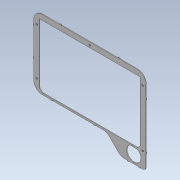
# Autodesk Inventor part: Лицевой лист
Saved by Autodesk Inventor 2021.2 (Build 252289000, 289)
## iProperties
Created: 2022-11-29
Part Number: Лицевой лист
Material: Типовые
Document SubType Name: ЛистМат
Designer: Voodoo
Density: 1 g/cm^3
Sheet Metal Rule: По умолчанию_мм
Appearance: По умолчанию
Mass: 42.3344 g
Surface Area: 479.036 cm^2
Volume: 42.3344 cm^3
Flat Pattern Width: 29.78 cm
Flat Pattern Length: 39.68 cm
Flat Pattern Area: 1181.67 cm^2
Sheet Metal Width: 297,800 мм
Sheet Metal Length: 396,800 мм
Sheet Metal Area: 118167,040 мм^2
Author: Voodoo
Autodesk Inventor part; units mm, degrees
ref_plane "YZ Plane" through (0, 0, 0) normal (1, 0, 0) x (0, 1, 0)
ref_plane "XZ Plane" through (0, 0, 0) normal (0, 1, 0) x (-1, 0, 0)
ref_plane "XY Plane" through (0, 0, 0) normal (0, 0, 1) x (1, 0, 0)
sketch "Эскиз6" plane through (0, 0, 2) normal (0, 0, 1) x (1, 0, 0)
  line L0 (-177, -106.1) -> (-177, 103.9)
  line L1 (-177, 103.9) -> (177, 103.9)
  line L2 (177, 103.9) -> (177, -106.1)
  line L3 (177, -106.1) -> (167, -116.1)
  line L4 (167, -116.1) -> (-167, -116.1)
  line L5 (-167, -116.1) -> (-177, -106.1)
  arc A0 (196.4, 92) -> (166.5, 121.9) centre (166.5, 92) ccw
  line L6 (-166.5, 121.9) -> (166.5, 121.9)
  arc A1 (-166.5, 121.9) -> (-196.4, 92) centre (-166.5, 92) ccw
  line L7 (-196.4, -92) -> (-196.4, 92)
  arc A2 (-196.4, -92) -> (-166.5, -121.9) centre (-166.5, -92) ccw
  line L8 (46.0736, -121.9) -> (-166.5, -121.9)
  arc A3 (68.7717, -131.3019) -> (46.0736, -121.9) centre (46.0736, -154) ccw
  line L9 (101.1981, -163.7283) -> (68.7717, -131.3019)
  arc A4 (101.1981, -163.7283) -> (120.9264, -171.9) centre (120.9264, -144) ccw
  line L10 (186.5, -171.9) -> (120.9264, -171.9)
  arc A5 (186.5, -171.9) -> (196.4, -162) centre (186.5, -162) ccw
  line L11 (196.4, 92) -> (196.4, -162)
  circle A6 centre (154.4, -141.9) radius 25
  line L12 (188.45, -115.4278) -> (188.45, -118.3722)
  line L13 (188.45, -118.3722) -> (185.9, -119.8445)
  line L14 (185.9, -119.8445) -> (183.35, -118.3722)
  line L15 (183.35, -118.3722) -> (183.35, -115.4278)
  line L16 (183.35, -115.4278) -> (185.9, -113.9555)
  line L17 (185.9, -113.9555) -> (188.45, -115.4278)
  line L18 (2.55, 112.8722) -> (2.55, 109.9278)
  line L19 (2.55, 109.9278) -> (0, 108.4555)
  line L20 (0, 108.4555) -> (-2.55, 109.9278)
  line L21 (-2.55, 109.9278) -> (-2.55, 112.8722)
  line L22 (-2.55, 112.8722) -> (0, 114.3445)
  line L23 (0, 114.3445) -> (2.55, 112.8722)
  line L24 (-183.35, 83.3722) -> (-183.35, 80.4278)
  line L25 (-183.35, 80.4278) -> (-185.9, 78.9555)
  line L26 (-185.9, 78.9555) -> (-188.45, 80.4278)
  line L27 (-188.45, 80.4278) -> (-188.45, 83.3722)
  line L28 (-188.45, 83.3722) -> (-185.9, 84.8445)
  line L29 (-185.9, 84.8445) -> (-183.35, 83.3722)
  line L30 (188.45, 83.3722) -> (188.45, 80.4278)
  line L31 (188.45, 80.4278) -> (185.9, 78.9555)
  line L32 (185.9, 78.9555) -> (183.35, 80.4278)
  line L33 (183.35, 80.4278) -> (183.35, 83.3722)
  line L34 (183.35, 83.3722) -> (185.9, 84.8445)
  line L35 (185.9, 84.8445) -> (188.45, 83.3722)
  line L36 (-183.35, -80.4278) -> (-183.35, -83.3722)
  line L37 (-183.35, -83.3722) -> (-185.9, -84.8445)
  line L38 (-185.9, -84.8445) -> (-188.45, -83.3722)
  line L39 (-188.45, -83.3722) -> (-188.45, -80.4278)
  line L40 (-188.45, -80.4278) -> (-185.9, -78.9555)
  line L41 (-185.9, -78.9555) -> (-183.35, -80.4278)
  line L42 (140.5306, -121.1) -> (168.2694, -121.1)
  point P0 (0, 0)
  dimension "d75" = 5
  measures "d75" distance between parallel lines of L4 L42
sketch "Эскиз7" plane through (0, 0, 0) normal (0, 0, -1) x (-1, 0, 0)
  line L0 (177, 103.9) -> (177, -106.1)
  line L1 (177, -106.1) -> (167, -116.1)
  line L2 (167, -116.1) -> (-167, -116.1)
  line L3 (-167, -116.1) -> (-177, -106.1)
  line L4 (-177, -106.1) -> (-177, 103.9)
  line L5 (-177, 103.9) -> (177, 103.9)
  line L6 (166.5, 121.9) -> (-166.5, 121.9)
  arc A0 (-166.5, 121.9) -> (-196.4, 92) centre (-166.5, 92) ccw
  line L7 (-196.4, 92) -> (-196.4, -162)
  arc A1 (-196.4, -162) -> (-186.5, -171.9) centre (-186.5, -162) ccw
  line L8 (-186.5, -171.9) -> (-120.9264, -171.9)
  arc A2 (-120.9264, -171.9) -> (-101.1981, -163.7283) centre (-120.9264, -144) ccw
  line L9 (-101.1981, -163.7283) -> (-68.7717, -131.3019)
  arc A3 (-46.0736, -121.9) -> (-68.7717, -131.3019) centre (-46.0736, -154) ccw
  line L10 (-46.0736, -121.9) -> (166.5, -121.9)
  arc A4 (166.5, -121.9) -> (196.4, -92) centre (166.5, -92) ccw
  line L11 (196.4, -92) -> (196.4, 92)
  arc A5 (196.4, 92) -> (166.5, 121.9) centre (166.5, 92) ccw
  arc A6 (-168.2694, -121.1) -> (-140.5306, -121.1) centre (-154.4, -141.9) ccw
  line L12 (-140.5306, -121.1) -> (-168.2694, -121.1)
  line L13 (-188.45, -118.3722) -> (-188.45, -115.4278)
  line L14 (-188.45, -115.4278) -> (-185.9, -113.9555)
  line L15 (-185.9, -113.9555) -> (-183.35, -115.4278)
  line L16 (-183.35, -115.4278) -> (-183.35, -118.3722)
  line L17 (-183.35, -118.3722) -> (-185.9, -119.8445)
  line L18 (-185.9, -119.8445) -> (-188.45, -118.3722)
  line L19 (-2.55, 109.9278) -> (-2.55, 112.8722)
  line L20 (-2.55, 112.8722) -> (0, 114.3445)
  line L21 (0, 114.3445) -> (2.55, 112.8722)
  line L22 (2.55, 112.8722) -> (2.55, 109.9278)
  line L23 (2.55, 109.9278) -> (0, 108.4555)
  line L24 (0, 108.4555) -> (-2.55, 109.9278)
  line L25 (183.35, 80.4278) -> (183.35, 83.3722)
  line L26 (183.35, 83.3722) -> (185.9, 84.8445)
  line L27 (185.9, 84.8445) -> (188.45, 83.3722)
  line L28 (188.45, 83.3722) -> (188.45, 80.4278)
  line L29 (188.45, 80.4278) -> (185.9, 78.9555)
  line L30 (185.9, 78.9555) -> (183.35, 80.4278)
  line L31 (-188.45, 80.4278) -> (-188.45, 83.3722)
  line L32 (-188.45, 83.3722) -> (-185.9, 84.8445)
  line L33 (-185.9, 84.8445) -> (-183.35, 83.3722)
  line L34 (-183.35, 83.3722) -> (-183.35, 80.4278)
  line L35 (-183.35, 80.4278) -> (-185.9, 78.9555)
  line L36 (-185.9, 78.9555) -> (-188.45, 80.4278)
  line L37 (183.35, -83.3722) -> (183.35, -80.4278)
  line L38 (183.35, -80.4278) -> (185.9, -78.9555)
  line L39 (185.9, -78.9555) -> (188.45, -80.4278)
  line L40 (188.45, -80.4278) -> (188.45, -83.3722)
  line L41 (188.45, -83.3722) -> (185.9, -84.8445)
  line L42 (185.9, -84.8445) -> (183.35, -83.3722)
  line L43 (-105, 121.9) -> (-100, 121.9)
  line L44 (-100, 121.9) -> (-100, 123.9)
  line L45 (-100, 123.9) -> (-105, 123.9)
  line L46 (-105, 123.9) -> (-105, 121.9)
  line L47 (100, 121.9) -> (105, 121.9)
  line L48 (105, 121.9) -> (105, 123.9)
  line L49 (105, 123.9) -> (100, 123.9)
  line L50 (100, 123.9) -> (100, 121.9)
  line L51 (0, 103.9) -> (0, 81.7755) construction
  line L52 (-196.4, 50) -> (-198.4, 50)
  line L53 (-198.4, 50) -> (-198.4, 45)
  line L54 (-198.4, 45) -> (-196.4, 45)
  line L55 (-196.4, 45) -> (-196.4, 50)
  line L56 (-196.4, -115) -> (-198.4, -115)
  line L57 (-198.4, -115) -> (-198.4, -120)
  line L58 (-198.4, -120) -> (-196.4, -120)
  line L59 (-196.4, -120) -> (-196.4, -115)
  line L60 (-176.4, -171.9) -> (-171.4, -171.9)
  line L61 (-171.4, -171.9) -> (-171.4, -173.9)
  line L62 (-171.4, -173.9) -> (-176.4, -173.9)
  line L63 (-176.4, -173.9) -> (-176.4, -171.9)
  line L64 (-18.6, -121.9) -> (-13.6, -121.9)
  line L65 (-13.6, -121.9) -> (-13.6, -123.9)
  line L66 (-13.6, -123.9) -> (-18.6, -123.9)
  line L67 (-18.6, -123.9) -> (-18.6, -121.9)
  line L68 (131.4, -121.9) -> (136.4, -121.9)
  line L69 (136.4, -121.9) -> (136.4, -123.9)
  line L70 (136.4, -123.9) -> (131.4, -123.9)
  line L71 (131.4, -123.9) -> (131.4, -121.9)
  line L72 (196.4, -28.1) -> (198.4, -28.1)
  line L73 (198.4, -28.1) -> (198.4, -23.1)
  line L74 (198.4, -23.1) -> (196.4, -23.1)
  line L75 (196.4, -23.1) -> (196.4, -28.1)
  line L76 (196.4, 76.9) -> (198.4, 76.9)
  line L77 (198.4, 76.9) -> (198.4, 71.9)
  line L78 (198.4, 71.9) -> (196.4, 71.9)
  line L79 (196.4, 71.9) -> (196.4, 76.9)
  line L80 (-196.4, -35) -> (-297.2205, -35)
  line L81 (-131.4, -171.9) -> (-136.4, -171.9)
  line L82 (-136.4, -171.9) -> (-136.4, -173.9)
  line L83 (-136.4, -173.9) -> (-131.4, -173.9)
  line L84 (-131.4, -173.9) -> (-131.4, -171.9)
  point P0 (0, 0)
  dimension "d81" = 5
  dimension "d82" = 2
  dimension "d83" = 5
  dimension "d84" = 2
  dimension "d85" = 100
  dimension "d86" = 100
  dimension "d87" = 2
  dimension "d88" = 5
  dimension "d89" = 2
  dimension "d90" = 5
  dimension "d91" = 5
  dimension "d92" = 2
  dimension "d93" = 5
  dimension "d94" = 2
  dimension "d95" = 5
  dimension "d96" = 2
  dimension "d97" = 2
  dimension "d98" = 5
  dimension "d99" = 2
  dimension "d100" = 5
  dimension "d101" = 80
  dimension "d102" = 80
  dimension "d103" = 20
  dimension "d104" = 60
  dimension "d105" = 150
  dimension "d106" = 45
  dimension "d107" = 100
  dimension "d113" = 5
  dimension "d114" = 2
  dimension "d115" = 40
  measures "d81" distance of L44.end L45.end
  measures "d82" distance of L45.end L43.start
  measures "d83" distance of L48.end L49.end
  measures "d84" distance of L49.end L47.start
  measures "d85" distance between parallel lines of L50 L51
  measures "d86" horizontal distance of L51.start L44.end
  measures "d87" distance of L54.end L53.end
  measures "d88" distance of L53.end L52.end
  measures "d89" distance of L58.end L57.end
  measures "d90" distance of L57.end L56.end
  measures "d91" distance of L61.end L62.end
  measures "d92" distance of L60.end L61.end
  measures "d93" distance of L65.end L66.end
  measures "d94" distance of L64.end L65.end
  measures "d95" distance of L69.end L70.end
  measures "d96" distance of L68.end L69.end
  measures "d97" distance of L74.end L73.end
  measures "d98" distance of L73.end L72.end
  measures "d99" distance of L77.end L78.end
  measures "d100" distance of L76.end L77.end
  measures "d101" distance between parallel lines of L56 L80
  measures "d102" distance from line of L54.end L80
  measures "d103" distance from line of L62.end L7
  measures "d104" distance from line of L69.end L11
  measures "d105" distance of L65.end L69.end
  measures "d106" distance from line of L76.end L6
  measures "d107" distance of L74.end L76.start
  measures "d113" distance of L83.end L82.end
  measures "d114" distance of L82.end L81.end
  measures "d115" distance from line of L63 L82.end
sketch "Эскиз1" plane through (0, 0, 0) normal (0, 0, 1) x (1, 0, 0)
  line L0 (-166.5, -124) -> (46.0736, -124)
  line L1 (198.5, -124) -> (198.5, 92)
  line L2 (166.5, 124) -> (-166.5, 124)
  line L3 (-198.5, 92) -> (-198.5, -92)
  line L4 (-198.5, -124) -> (198.5, 124) construction
  line L5 (198.5, -124) -> (-198.5, 124) construction
  arc A0 (-166.5, 124) -> (-198.5, 92) centre (-166.5, 92) ccw
  arc A1 (198.5, 92) -> (166.5, 124) centre (166.5, 92) ccw
  arc A2 (-198.5, -92) -> (-166.5, -124) centre (-166.5, -92) ccw
  line L6 (198.5, -124) -> (198.5, -162)
  line L7 (186.5, -174) -> (120.9264, -174)
  line L8 (99.7132, -165.2132) -> (67.2868, -132.7868)
  arc A3 (186.5, -174) -> (198.5, -162) centre (186.5, -162) ccw
  arc A4 (99.7132, -165.2132) -> (120.9264, -174) centre (120.9264, -144) ccw
  arc A5 (67.2868, -132.7868) -> (46.0736, -124) centre (46.0736, -154) ccw
  line L9 (-166.5, 121.9) -> (166.5, 121.9)
  arc A6 (196.4, 92) -> (166.5, 121.9) centre (166.5, 92) ccw
  line L10 (196.4, 92) -> (196.4, -145)
  line L11 (196.4, -145) -> (196.4, -162)
  arc A7 (186.5, -171.9) -> (196.4, -162) centre (186.5, -162) ccw
  line L12 (186.5, -171.9) -> (120.9264, -171.9)
  arc A8 (101.1981, -163.7283) -> (120.9264, -171.9) centre (120.9264, -144) ccw
  line L13 (101.1981, -163.7283) -> (68.7717, -131.3019)
  arc A9 (68.7717, -131.3019) -> (46.0736, -121.9) centre (46.0736, -154) ccw
  line L14 (46.0736, -121.9) -> (-166.5, -121.9)
  arc A10 (-196.4, -92) -> (-166.5, -121.9) centre (-166.5, -92) ccw
  line L15 (-196.4, -92) -> (-196.4, 92)
  arc A11 (-166.5, 121.9) -> (-196.4, 92) centre (-166.5, 92) ccw
  point P0 (0, 0)
  point P1 (198.5, -174)
  point P2 (108.5, -174)
  dimension "d2" = 397
  dimension "d3" = 248
  dimension "d4" = 32
  dimension "d5" = 298
  dimension "d6" = 12
  dimension "d7" = 50
  dimension "d8" = 90
  dimension "d9" = 135
  dimension "d10" = 30
  dimension "d11" = 2.1
  constraints: 32 end point, 24 point on circle, 12 centre point, 12 point on line, 12 tangent, 4 parallel, 4 perpendicular, 3 equal radius, 2 midpoint, 1 horizontal, 12 other
  measures "d2" distance of L5.end L4.end
  measures "d3" distance of L4.end L1.start
  measures "d4" radius of A0
  measures "d5" distance between parallel lines of L7 L2
  measures "d6" radius of A3
  measures "d7" distance between parallel lines of L0 L7
  measures "d8" distance from line of L6 point (108.5, -174)
  measures "d9" angle of L0 L8
  measures "d10" radius of A4
  measures "d11" distance between parallel lines of L2 L9
extrude "Пластина1" add sketch "Эскиз1" along normal blind 2 contours L9 A6 L10 L11 A7 L12 A8 L13 A9 L14 A10 L15 A11
sketch "Эскиз3" plane through (0, 0, 0) normal (0, 0, -1) x (-1, 0, 0)
  line L0 (166.5, 121.9) -> (-166.5, 121.9) projected
  arc A0 (-166.5, 121.9) -> (-196.4, 92) centre (-166.5, 92) ccw projected
  line L1 (-196.4, 92) -> (-196.4, -162) projected
  arc A1 (-196.4, -162) -> (-186.5, -171.9) centre (-186.5, -162) ccw projected
  line L2 (-186.5, -171.9) -> (-120.9264, -171.9) projected
  arc A2 (-120.9264, -171.9) -> (-101.1981, -163.7283) centre (-120.9264, -144) ccw projected
  line L3 (-101.1981, -163.7283) -> (-68.7717, -131.3019) projected
  arc A3 (-46.0736, -121.9) -> (-68.7717, -131.3019) centre (-46.0736, -154) ccw projected
  line L4 (-46.0736, -121.9) -> (166.5, -121.9) projected
  arc A4 (166.5, -121.9) -> (196.4, -92) centre (166.5, -92) ccw projected
  line L5 (196.4, -92) -> (196.4, 92) projected
  arc A5 (196.4, 92) -> (166.5, 121.9) centre (166.5, 92) ccw projected
  circle A6 centre (-154.4, -141.9) radius 25
  point P0 (0, 0)
  dimension "d19" = 50
  dimension "d20" = 30
  dimension "d21" = 42
  constraints: 1 centre point
  measures "d19" diameter of A6
  measures "d20" distance from line of A6.centre L2
  measures "d21" distance from line of A6.centre L1
extrude "Вырез2" cut sketch "Эскиз3" against normal blind 2 contours A6
sketch "Эскиз4" plane through (0, 0, 2) normal (0, 0, 1) x (1, 0, 0)
  circle A0 centre (154.4, -141.9) radius 25 projected
  arc A1 (196.4, 92) -> (166.5, 121.9) centre (166.5, 92) ccw projected
  line L0 (-166.5, 121.9) -> (166.5, 121.9) projected
  arc A2 (-166.5, 121.9) -> (-196.4, 92) centre (-166.5, 92) ccw projected
  line L1 (-196.4, -92) -> (-196.4, 92) projected
  arc A3 (-196.4, -92) -> (-166.5, -121.9) centre (-166.5, -92) ccw projected
  line L2 (46.0736, -121.9) -> (-166.5, -121.9) projected
  arc A4 (68.7717, -131.3019) -> (46.0736, -121.9) centre (46.0736, -154) ccw projected
  line L3 (101.1981, -163.7283) -> (68.7717, -131.3019) projected
  arc A5 (101.1981, -163.7283) -> (120.9264, -171.9) centre (120.9264, -144) ccw projected
  line L4 (186.5, -171.9) -> (120.9264, -171.9) projected
  arc A6 (186.5, -171.9) -> (196.4, -162) centre (186.5, -162) ccw projected
  line L5 (196.4, 92) -> (196.4, -162) projected
  circle A7 centre (-185.9, -81.9) radius 2.1
  circle A8 centre (-185.9, 81.9) radius 2.1
  circle A9 centre (0, 111.4) radius 2.1
  circle A10 centre (185.9, 81.9) radius 2.1
  circle A11 centre (185.9, -116.9) radius 2.1
  line L6 (-183.35, 80.4278) -> (-185.9, 78.9555)
  line L7 (-185.9, 78.9555) -> (-188.45, 80.4278)
  line L8 (-188.45, 80.4278) -> (-188.45, 83.3722)
  line L9 (-188.45, 83.3722) -> (-185.9, 84.8445)
  line L10 (-185.9, 84.8445) -> (-183.35, 83.3722)
  line L11 (-183.35, 83.3722) -> (-183.35, 80.4278)
  line L12 (2.55, 109.9278) -> (0, 108.4555)
  line L13 (0, 108.4555) -> (-2.55, 109.9278)
  line L14 (-2.55, 109.9278) -> (-2.55, 112.8722)
  line L15 (-2.55, 112.8722) -> (0, 114.3445)
  line L16 (0, 114.3445) -> (2.55, 112.8722)
  line L17 (2.55, 112.8722) -> (2.55, 109.9278)
  line L18 (188.45, 80.4278) -> (185.9, 78.9555)
  line L19 (185.9, 78.9555) -> (183.35, 80.4278)
  line L20 (183.35, 80.4278) -> (183.35, 83.3722)
  line L21 (183.35, 83.3722) -> (185.9, 84.8445)
  line L22 (185.9, 84.8445) -> (188.45, 83.3722)
  line L23 (188.45, 83.3722) -> (188.45, 80.4278)
  line L24 (188.45, -118.3722) -> (185.9, -119.8445)
  line L25 (185.9, -119.8445) -> (183.35, -118.3722)
  line L26 (183.35, -118.3722) -> (183.35, -115.4278)
  line L27 (183.35, -115.4278) -> (185.9, -113.9555)
  line L28 (185.9, -113.9555) -> (188.45, -115.4278)
  line L29 (188.45, -115.4278) -> (188.45, -118.3722)
  line L30 (-183.35, -83.3722) -> (-185.9, -84.8445)
  line L31 (-185.9, -84.8445) -> (-188.45, -83.3722)
  line L32 (-188.45, -83.3722) -> (-188.45, -80.4278)
  line L33 (-188.45, -80.4278) -> (-185.9, -78.9555)
  line L34 (-185.9, -78.9555) -> (-183.35, -80.4278)
  line L35 (-183.35, -80.4278) -> (-183.35, -83.3722)
  point P0 (0, 0)
  point P1 (0, 121.9)
  dimension "d34" = 4.2
  dimension "d36" = 4.2
  dimension "d37" = 4.2
  dimension "d38" = 4.2
  dimension "d52" = 5.1
  dimension "d53" = 5.1
  dimension "d54" = 5.1
  dimension "d55" = 5.1
  dimension "d56" = 5.1
  dimension "d57" = 10.5
  dimension "d58" = 10.5
  dimension "d59" = 10.5
  dimension "d60" = 10.5
  dimension "d61" = 55
  dimension "d62" = 40
  dimension "d63" = 40
  dimension "d64" = 4.2
  dimension "d65" = 10.5
  constraints: 60 end point, 6 vertical alignment, 5 centre point, 5 coincident, 1 horizontal alignment, 1 midpoint, 65 other
  measures "d34" diameter of A7
  measures "d36" diameter of A9
  measures "d37" diameter of A10
  measures "d38" diameter of A11
  measures "d52" distance between parallel lines of L11 L8
  measures "d53" distance between parallel lines of L17 L14
  measures "d54" distance between parallel lines of L20 L23
  measures "d55" distance between parallel lines of L29 L26
  measures "d56" distance between parallel lines of L35 L32
  measures "d57" distance from line of L5 A10.centre
  measures "d58" distance from line of A9.centre L0
  measures "d59" distance from line of point (-185.9, 81.9) L1
  measures "d60" distance from line of A7.centre L1
  measures "d61" distance from line of A11.centre L4
  measures "d62" distance from line of L0 A8.centre
  measures "d63" distance from line of L2 point (-185.9, -81.9)
  measures "d64" diameter of A8
  measures "d65" distance from line of L5 point (185.9, -116.9)
extrude "Вырез3" cut sketch "Эскиз4" against normal blind 2 contours L6 L7 L8 L9 L10 L11 | L12 L13 L14 L15 L16 L17 | L18 L19 L20 L21 L22 L23 | L24 L25 L26 L27 L28 L29 | L30 L31 L32 L33 L34 L35
sketch "Эскиз5" plane through (0, 0, 2) normal (0, 0, 1) x (1, 0, 0)
  line L0 (-177, 103.9) -> (177, 103.9)
  line L1 (177, 103.9) -> (177, -106.1)
  line L2 (167, -116.1) -> (-167, -116.1)
  line L3 (-177, -106.1) -> (-177, 103.9)
  line L4 (-166.5, 121.9) -> (166.5, 121.9) projected
  line L5 (-177, -106.1) -> (-167, -116.1)
  line L6 (167, -116.1) -> (177, -106.1)
  point P0 (0, 0)
  point P1 (177, -116.1)
  point P2 (-177, -116.1)
  point P3 (0, 103.9)
  point P4 (0, 121.9)
  dimension "d66" = 354
  dimension "d67" = 220
  dimension "d68" = 18
  dimension "d69" = 10
  dimension "d70" = 10
  dimension "d71" = 10
  dimension "d72" = 10
  constraints: 12 end point, 4 point on line, 2 midpoint, 2 parallel, 1 horizontal, 1 perpendicular, 1 vertical alignment
  measures "d66" distance of L0.start L0.end
  measures "d67" distance of point (-177, -116.1) L0.start
  measures "d68" distance between parallel lines of L4 L0
  measures "d69" distance of L3.start point (-177, -116.1)
  measures "d70" distance of L2.end point (-177, -116.1)
  measures "d71" distance of L2.start point (177, -116.1)
  measures "d72" distance of L1.end point (177, -116.1)
extrude "Вырез4" cut sketch "Эскиз5" against normal blind 2
sheet face with bend "Грань2" sketch "Эскиз6" thickness 2 toward (0, 0, -1) bend radius 2 picked at (151.5202, -120.2134) contours L42 A6
bend "Сгиб1"
sheet face with bend "Грань3" sketch "Эскиз7" thickness 2 toward (0, 0, 1) bend radius 2 contours L6 L50 L49 L48 | L76 L77 L78 L11 | L6 L46 L45 L44 | L74 L73 L72 L11 | L7 L54 L53 L52 | L69 L70 L71 L10 | L7 L58 L57 L56 | L65 L66 L67 L10 | L8 L61 L62 L63 | L8 L84 L83 L82
bend "Сгиб2"
equation "\"d22\" = Толщина"
equation "\"d34\" = d35"
equation "\"d36\" = d35"
equation "\"d37\" = d36"
equation "\"d38\" = d37"
equation "\"d54\" = d53"
equation "\"d55\" = d54"
equation "\"d56\" = d52"
equation "\"d59\" = d60"
equation "\"d60\" = d57"
equation "\"d65\" = d57"
equation "\"d50\" = Толщина"
equation "\"d70\" = d69"
equation "\"d71\" = d69"
equation "\"d72\" = d71"
equation "\"d73\" = Толщина"
equation "\"d86\" = d85"
equation "\"d102\" = d101"
equation "\"d12\" = Толщина"
equation "\"d76\" = Радиус_гибки"
equation "\"d77\" = Ширина_просечки"
equation "\"d79\" = Мин_остаток"
equation "\"d78\" = Глубина_просечки"
equation "\"d80\" = Радиус_перехода"
equation "\"d108\" = Радиус_гибки"
equation "\"d109\" = Ширина_просечки"
equation "\"d111\" = Мин_остаток"
equation "\"d110\" = Глубина_просечки"
equation "\"d112\" = Радиус_перехода"
equation "\"Радиус_гибки\" = Толщина"
equation "\"Ширина_просечки\" = Толщина"
equation "\"Глубина_просечки\" = 0.5 * Толщина"
equation "\"Размер_просечки\" = 4 * Толщина"
equation "\"Мин_остаток\" = 2 * Толщина"
equation "\"Радиус_перехода\" = Радиус_гибки"
equation "\"Радиус_Якоби\" = Радиус_гибки"
equation "\"Размер_зазора\" = Толщина"
equation "\"Толщина\" = 2"
equation "\"d35\" = 4.2"
